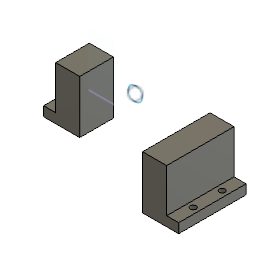
servo holder (Autodesk Fusion 360 design; units mm, degrees)
part number: 2026-03-16-18-08-13-448
Autodesk Fusion 360 part; units mm, degrees
sketch "Sketch2" plane through (0, 5, 0) normal (0, 1, 0) x (-1, 0, 0)
  line L0 (-160, 0) -> (0, 0)
  line L1 (0, 0) -> (0, 160)
  line L2 (0, 160) -> (-160, 160)
  line L3 (-160, 160) -> (-160, 0)
  line L4 (-160, 80) -> (0, 80)
  line L5 (0, 80) -> (-160, 80)
  line L6 (-160, 80) -> (-160, 92)
  line L7 (-160, 92) -> (0, 92)
  line L8 (0, 92) -> (0, 80)
  line L9 (0, 92) -> (-60, 92)
  line L10 (-60, 92) -> (-60, 120)
  line L11 (-60, 120) -> (0, 120)
  line L12 (0, 120) -> (0, 92)
  line L13 (-160, 92) -> (-100, 92)
  line L14 (-100, 92) -> (-100, 120)
  line L15 (-100, 120) -> (-160, 120)
  line L16 (-160, 120) -> (-160, 92)
  line L17 (-60, 92) -> (-50, 92)
  line L18 (-50, 92) -> (-50, 120)
  line L19 (-50, 120) -> (-60, 120)
  line L20 (-60, 120) -> (-60, 92)
  line L21 (-100, 92) -> (-110, 92)
  line L22 (-110, 92) -> (-110, 120)
  line L23 (-110, 120) -> (-100, 120)
  line L24 (-100, 120) -> (-100, 92)
  dimension "d7" = 160
  dimension "d8" = 12
  dimension "d9" = 60
  dimension "d10" = 28
  dimension "d11" = 60
  dimension "d12" = 28
  dimension "d13" = 10
  dimension "d14" = 28
  dimension "d15" = 10
  dimension "d16" = 28
  constraint midpoint L3 L4.start
  constraint midpoint L1 L4.end
  constraint horizontal L5
  constraint vertical L6
  constraint horizontal L7
  constraint vertical L8
  constraint horizontal L9
  constraint vertical L10
  constraint horizontal L11
  constraint vertical L12
  constraint horizontal L13
  constraint vertical L14
  constraint horizontal L15
  constraint vertical L16
  constraint horizontal L17
  constraint vertical L18
  constraint horizontal L19
  constraint vertical L20
  constraint horizontal L21
  constraint vertical L22
  constraint horizontal L23
  constraint vertical L24
  measures "d7" distance of L4.end L4.start
  measures "d8" distance of L4.end L7.end
  measures "d9" distance of L7.end L9.end
  measures "d10" distance of L7.end L11.end
  measures "d11" distance of L6.end L13.end
  measures "d12" distance of L6.end L15.end
  measures "d13" distance of L9.end L17.end
  measures "d14" distance of L9.end L10.end
  measures "d15" distance of L13.end L21.end
  measures "d16" distance of L13.end L14.end
extrude "Extrude2" add sketch "Sketch2" along normal blind 22 contours L7 L13 L14 L15 L21 L22 L23 L24 | L7 L9 L10 L11 L17 L18 L19 L20 makes body 1 at (60, 12.3333, 101.3333) makes body 2 at (110, 12.3333, 101.3333)
sketch "Sketch3" plane through (0, 0, 92) normal (0, 0, -1) x (-1, 0, 0)
  line L0 (-100, 5) -> (-100, 27)
  line L1 (-100, 27) -> (-110, 27)
  line L2 (-110, 27) -> (-110, 5)
  line L3 (-105, 5) -> (-105, 7.3)
  circle A0 centre (-105, 9.45) radius 2.15
  circle A1 centre (-105.1004, 19.2477) radius 2.15
  line L4 (-105, 9.45) -> (-105.1004, 19.2477)
  line L5 (-55, 5) -> (-55, 7.3)
  circle A2 centre (-55, 9.45) radius 2.15
  line L6 (-55, 9.45) -> (-55, 19.248)
  circle A3 centre (-55, 19.248) radius 2.15
  circle A4 centre (-105.1004, 19.2477) radius 0.9
  circle A5 centre (-105, 9.45) radius 0.9
  circle A6 centre (-55, 9.45) radius 0.9
  circle A7 centre (-55, 19.248) radius 0.9
  line L7 (-110, 5) -> (-100, 5)
  dimension "d19" = 2.3
  dimension "d20" = 2.15
  dimension "d23" = 2.3
  dimension "d24" = 2.15
  dimension "d26" = 9.798
  dimension "d27" = 4.3
  dimension "d28" = 1.8
  dimension "d29" = 1.8
  dimension "d30" = 1.8
  dimension "d31" = 1.8
  constraint coincident L3.end A0
  constraint coincident A0.centre L4.start
  constraint coincident A1.centre L4.end
  constraint vertical L5
  constraint coincident L5.end A2
  constraint coincident A2.centre L6.start
  constraint vertical L6
  constraint coincident L6.end A3.centre
  constraint concentric A1 A4
  constraint concentric A0 A5
  constraint concentric A2 A6
  constraint concentric A3 A7
  measures "d19" distance of L3.start L3.end
  measures "d20" distance of L3.end A0.centre
  measures "d23" distance of L5.start L5.end
  measures "d24" distance of L5.end A2.centre
  measures "d26" distance of A2.centre L6.end
  measures "d27" diameter of A3
  measures "d28" diameter of A4
  measures "d29" diameter of A5
  measures "d30" diameter of A6
  measures "d31" diameter of A7
extrude "Extrude3" cut sketch "Sketch3" against normal blind 10 contours A4 | A5 | A6 | A7 bodies 1 2
sketch "Sketch4" plane through (0, 0, 92) normal (0, 0, -1) x (-1, 0, 0)
  circle A0 centre (-55, 9.45) radius 0.9
  circle A1 centre (-55, 19.248) radius 0.9
  line L0 (-50, 5) -> (-50, 27)
  line L1 (-50, 27) -> (-60, 27)
  line L2 (-60, 27) -> (-60, 5)
  line L3 (-60, 5) -> (-50, 5)
  circle A2 centre (-69, 13.3) radius 2.9
  dimension "d37" = 5.8
  measures "d37" diameter of A2
sketch "Sketch5" plane through (0, 0, 0) normal (0, 1, 0) x (1, 0, 0)
  line L0 (60, -120) -> (60, -92)
  line L1 (60, -92) -> (50, -92)
  line L2 (50, -92) -> (50, -120)
  line L3 (50, -120) -> (60, -120)
  line L4 (100, -120) -> (110, -120)
  line L5 (110, -120) -> (110, -92)
  line L6 (110, -92) -> (100, -92)
  line L7 (100, -92) -> (100, -120)
  line L8 (95, -92) -> (100, -92)
  line L9 (100, -92) -> (100, -120)
  line L10 (110, -120) -> (115, -120)
  line L11 (115, -120) -> (115, -92)
  line L12 (115, -92) -> (110, -92)
  line L13 (110, -92) -> (110, -120)
  line L14 (100, -120) -> (95, -120)
  line L15 (95, -120) -> (95, -92)
  line L16 (95, -92) -> (100, -92)
  line L17 (100, -92) -> (100, -120)
  line L18 (60, -120) -> (65, -120)
  line L19 (65, -120) -> (65, -92)
  line L20 (65, -92) -> (60, -92)
  line L21 (60, -92) -> (60, -120)
  line L22 (50, -120) -> (45, -120)
  line L23 (45, -120) -> (45, -92)
  line L24 (45, -92) -> (50, -92)
  line L25 (50, -92) -> (50, -120)
  dimension "d40" = 28
  dimension "d41" = 5
  dimension "d42" = 28
  dimension "d43" = 5
  dimension "d44" = 5
  dimension "d45" = 28
  dimension "d46" = 5
  dimension "d47" = 28
  constraint horizontal L8
  constraint vertical L9
  constraint coincident L4.start L7.end
  constraint horizontal L10
  constraint vertical L11
  constraint horizontal L12
  constraint vertical L13
  constraint coincident L4.end L5.start
  constraint horizontal L14
  constraint vertical L15
  constraint horizontal L16
  constraint vertical L17
  constraint horizontal L18
  constraint vertical L19
  constraint horizontal L20
  constraint vertical L21
  constraint coincident L0.start L3.end
  constraint horizontal L22
  constraint vertical L23
  constraint horizontal L24
  constraint vertical L25
  constraint coincident L2.end L3.start
  measures "d40" distance of L4.start L6.end
  measures "d41" distance of L4.end L10.end
  measures "d42" distance of L4.end L5.end
  measures "d43" distance of L4.start L14.end
  measures "d44" distance of L0.start L18.end
  measures "d45" distance of L0.start L0.end
  measures "d46" distance of L2.end L22.end
  measures "d47" distance of L2.end L1.end
move_body "Move1" bodies 1 2 to x (1, 0, 0) y (0, 1, 0) z (0, 0, 1) at (0, -5, 0)
extrude "Extrude5" add sketch "Sketch5" along normal blind 4 contours L0 L18 L19 L20 L21 | L2 L22 L23 L24 L25 | L7 L8 L9 L14 L15 L16 L17 | L5 L10 L11 L12 L13 bodies 1 2
sketch "Sketch6" plane through (0, 4, 0) normal (0, 1, 0) x (-1, 0, 0)
  line L0 (-100, 92) -> (-95, 92)
  line L1 (-95, 92) -> (-95, 120)
  line L2 (-95, 120) -> (-100, 120)
  line L3 (-100, 120) -> (-100, 92)
  circle A0 centre (-97.5136, 111.5) radius 1.2
  circle A1 centre (-97.5136, 99.5) radius 1.2
  circle A2 centre (-112.5136, 111.5) radius 1.2
  circle A3 centre (-112.5136, 99.5) radius 1.2
  circle A4 centre (-47.5136, 111.5) radius 1.2
  circle A5 centre (-62.5136, 111.5) radius 1.2
  circle A6 centre (-62.5136, 99.5) radius 1.2
  circle A7 centre (-47.5136, 99.5) radius 1.2
  dimension "d54" = 2.4
  dimension "d55" = 2.4
  dimension "d56" = 2.4
  dimension "d57" = 2.4
  dimension "d58" = 2.4
  dimension "d59" = 2.4
  dimension "d60" = 2.4
  dimension "d61" = 2.4
  measures "d54" diameter of A0
  measures "d55" diameter of A1
  measures "d56" diameter of A2
  measures "d57" diameter of A3
  measures "d58" diameter of A4
  measures "d59" diameter of A7
  measures "d60" diameter of A5
  measures "d61" diameter of A6
extrude "Extrude6" cut sketch "Sketch6" against normal blind 10 contours A0 | A1 | A2 | A3 | A4 | A5 | A6 | A7 bodies 1 2
sketch "Sketch7" plane through (0, 0, 92) normal (0, 0, -1) x (-1, 0, 0)
  circle A0 centre (-105, 4.45) radius 0.9
  circle A1 centre (-105.1004, 14.2477) radius 0.9
  line L0 (-115, 0) -> (-95, 0)
  line L1 (-95, 0) -> (-95, 4)
  line L2 (-95, 4) -> (-100, 4)
  line L3 (-100, 4) -> (-100, 22)
  line L4 (-100, 22) -> (-110, 22)
  line L5 (-110, 22) -> (-110, 4)
  line L6 (-110, 4) -> (-115, 4)
  line L7 (-115, 4) -> (-115, 0)
  line L8 (-100, 4) -> (-60, 4)
  line L9 (-60, 4) -> (-60, 0)
  line L10 (-60, 0) -> (-100, 0)
  line L11 (-100, 0) -> (-100, 4)
  constraint horizontal L8
  constraint vertical L9
  constraint horizontal L10
  constraint vertical L11
  constraint coincident L2.end L3.start
extrude "Extrude7" cut sketch "Sketch7" against normal blind 100 contours L0 L1 L2 L8 L10 L11 | L1 L8 L9 L10 bodies 1 2
sketch "Sketch8" plane through (50, 0, 0) normal (-1, 0, 0) x (0, 0, 1)
  line L0 (92, 4) -> (120, 4)
  line L1 (120, 4) -> (120, 22)
  line L2 (120, 22) -> (92, 22)
  line L3 (92, 22) -> (92, 4)
  line L4 (92, 0) -> (106, 0)
  line L5 (106, 0) -> (106, 22)
  line L6 (106, 22) -> (92, 22)
  line L7 (92, 22) -> (92, 0)
  line L8 (106, 22) -> (120, 22)
  line L9 (120, 22) -> (120, 0)
  line L10 (120, 0) -> (106, 0)
  line L11 (106, 0) -> (106, 22)
  dimension "d66" = 14
  dimension "d67" = 22
  constraint horizontal L4
  constraint vertical L5
  constraint horizontal L6
  constraint vertical L7
  constraint horizontal L8
  constraint vertical L9
  constraint horizontal L10
  constraint vertical L11
  measures "d66" distance of L4.start L4.end
  measures "d67" distance of L4.start L2.end
extrude "Extrude8" cut sketch "Sketch8" along normal blind 17 and the other way blind 32 contours L0 L1 L2 L5 L8 L9 L11 | L0 L5 L9 L10 L11 bodies 1
